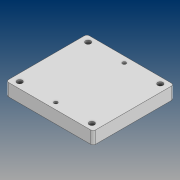
# Autodesk Inventor part: 23_Nap_hop_so_ngang
Saved by Autodesk Inventor 2021 (Build 250183000, 183)
## iProperties
Created: 2024-04-07
Part Number: 23_Nap_hop_so_ngang
Material: Generic
Document SubType Name: Modeling
Designer: Admin
Density: 1 g/cm^3
Appearance: Default
Author: Admin
Autodesk Inventor part; units mm, degrees
ref_plane "YZ Plane" through (0, 0, 0) normal (1, 0, 0) x (0, 1, 0)
ref_plane "XZ Plane" through (0, 0, 0) normal (0, 1, 0) x (-1, 0, 0)
ref_plane "XY Plane" through (0, 0, 0) normal (0, 0, 1) x (1, 0, 0)
sketch "Sketch1" plane through (0, 0, 0) normal (0, 1, 0) x (-1, 0, 0)
  line L0 (-35, 32.5) -> (35, 32.5)
  line L1 (35, 32.5) -> (35, -32.5)
  line L2 (35, -32.5) -> (-35, -32.5)
  line L3 (-35, -32.5) -> (-35, 32.5)
  line L4 (-35, 32.5) -> (35, -32.5) construction
  line L5 (35, 32.5) -> (-35, -32.5) construction
  line L6 (-35, 22.5) -> (35, 22.5)
  line L7 (35, 22.5) -> (35, -22.5)
  line L8 (35, -22.5) -> (-35, -22.5)
  line L9 (-35, -22.5) -> (-35, 22.5)
  line L10 (-35, 22.5) -> (35, -22.5) construction
  line L11 (35, 22.5) -> (-35, -22.5) construction
  point P0 (0, 0)
  dimension "d0" = 70
  dimension "d1" = 65
  dimension "d2" = 10
  constraints: 24 end point, 4 midpoint, 4 parallel, 2 horizontal, 2 perpendicular, 1 point on line
  measures "d0" distance of L1.end L2.end
  measures "d1" distance of L0.end L1.end
  measures "d2" distance between parallel lines of L2 L8
extrude "Extrusion1" add sketch "Sketch1" along normal blind 10
sketch "Sketch2" plane through (0, 0, 0) normal (0, -1, 0) x (1, 0, 0)
  line L0 (35, 32.5) -> (35, -32.5) projected
  line L1 (-35, 32.5) -> (35, 32.5) projected
  line L2 (-35, -32.5) -> (-35, 32.5) projected
  line L3 (35, -32.5) -> (-35, -32.5) projected
  line L4 (-35, 22.5) -> (35, 22.5)
  line L5 (35, 22.5) -> (35, -22.5)
  line L6 (35, -22.5) -> (-35, -22.5)
  line L7 (-35, -22.5) -> (-35, 22.5)
  line L8 (-35, 22.5) -> (35, -22.5) construction
  line L9 (35, 22.5) -> (-35, -22.5) construction
  line L10 (35, 32.5) -> (35, -32.5) projected
  line L11 (-35, -22.5) -> (35, -32.5) construction
  line L12 (0, -27.5) -> (29, -27.5) construction
  point P0 (0, 0)
  dimension "d5" = 10
  dimension "d6" = 6
  constraints: 16 end point, 3 midpoint, 2 parallel, 2 perpendicular, 1 horizontal, 1 point on line
  measures "d5" distance between parallel lines of L3 L6
  measures "d6" distance from line of L0 L12.end
hole "Hole1" at (29, 0, -27.5) direction (0, 1, 0) diameter 4.2 end through all counterbore diameter 8 counterbore depth 4
mirror "Mirror1" about plane through (0, 0, 0) normal (1, 0, 0) of "Hole1"
mirror "Mirror2" about plane through (0, 0, 0) normal (0, 0, 1) of "Hole1", "Mirror1"
fillet "Fillet1" radius 2 4 edges at (35, 5, 32.5) (-35, 5, 32.5) (-35, 5, -32.5) (35, 5, -32.5)
sketch "Sketch3" plane through (0, 0, 0) normal (0, -1, 0) x (1, 0, 0)
  arc A0 (33, -32.5) -> (35, -30.5) centre (33, -30.5) ccw projected
  line L0 (35, 30.5) -> (35, -30.5) projected
  arc A1 (35, 30.5) -> (33, 32.5) centre (33, 30.5) ccw projected
  line L1 (-33, 32.5) -> (33, 32.5) projected
  arc A2 (-33, 32.5) -> (-35, 30.5) centre (-33, 30.5) ccw projected
  line L2 (-35, -30.5) -> (-35, 30.5) projected
  arc A3 (-35, -30.5) -> (-33, -32.5) centre (-33, -30.5) ccw projected
  line L3 (33, -32.5) -> (-33, -32.5) projected
  circle A4 centre (-29, 27.5) radius 4 projected
  circle A5 centre (29, 27.5) radius 4 projected
  circle A6 centre (-29, -27.5) radius 4 projected
  circle A7 centre (29, -27.5) radius 4 projected
  circle A8 centre (29, 27.5) radius 2.1 projected
  circle A9 centre (-29, 27.5) radius 4 projected
  line L4 (29, 27.5) -> (-29, 27.5)
  circle A10 centre (29, -27.5) radius 2.1 projected
  line L5 (29, -27.5) -> (-29, -27.5)
  point P0 (0, 0)
  point P1 (0, 27.5)
  point P2 (0, -27.5)
  constraints: 4 end point, 2 horizontal, 2 midpoint
hole "Hole2" at (0, 0, 27.5) at (0, 0, -27.5) direction (0, 1, 0) diameter 2.8 end through all
body "Solid1"
